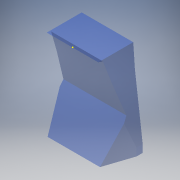
# Autodesk Inventor part: add
Saved by Autodesk Inventor 2018.1 (Build 221171000, 171)
## iProperties
Created: 2017-10-13
Part Number: add
Material: 一般
Document SubType Name: Modeling
Designer: kuwano
Density: 1 g/cm^3
Appearance: クリア - 青
Author: kuwano
Autodesk Inventor part; units mm, degrees
ref_plane "YZ Plane" through (0, 0, 0) normal (1, 0, 0) x (0, 1, 0)
ref_plane "XZ Plane" through (0, 0, 0) normal (0, 1, 0) x (-1, 0, 0)
ref_plane "XY Plane" through (0, 0, 0) normal (0, 0, 1) x (1, 0, 0)
sketch "スケッチ1" plane through (0, 0, 0) normal (0, 1, 0) x (-1, 0, 0)
  line L0 (341.5, 441.624) -> (-341.5, 441.624)
  line L1 (-341.5, 441.624) -> (-341.5, -441.624)
  line L2 (-341.5, -441.624) -> (341.5, -441.624)
  line L3 (341.5, -441.624) -> (341.5, 441.624)
  line L4 (0, -618.2736) -> (0, 618.2736) projected
  line L5 (478.1, 0) -> (-478.1, 0) projected
  point P0 (0, 0)
  point P1 (0, 441.624)
  point P2 (341.5, 0)
  dimension "d0" = 883.248
  dimension "d1" = 683
  constraints: 8 end point, 2 midpoint, 2 parallel, 2 point on line, 1 horizontal, 1 perpendicular
  measures "d0" distance of L2.end L0.start
  measures "d1" distance of L0.start L0.end
extrude "押し出し1" add sketch "スケッチ1" along normal blind 338.552
sketch "スケッチ2" plane through (0, 0, 0) normal (0, -1, 0) x (1, 0, 0)
  line L0 (-341.5, 441.624) -> (341.5, 441.624) projected
  line L1 (249.8123, 441.624) -> (266.1663, 220.287)
  line L2 (266.1663, 220.287) -> (341.5, -367.5482)
  line L3 (341.5, 441.624) -> (341.5, -441.624) projected
  line L4 (249.8123, 441.624) -> (341.5, 441.624)
  line L5 (341.5, 441.624) -> (341.5, -367.5482)
  line L6 (0, -782.4861) -> (0, 1603.5489) projected
  line L7 (-249.8123, 441.624) -> (-266.1663, 220.287)
  line L8 (-266.1663, 220.287) -> (-341.5, -367.5482)
  line L9 (-249.8123, 441.624) -> (-341.5, 441.624)
  line L10 (-341.5, 441.624) -> (-341.5, -367.5482)
  point P0 (0, 0)
  point P1 (0, 1262.6867)
  point P2 (-341.5, 441.624)
  constraints: 16 end point, 5 symmetric about line, 3 point on line, 1 horizontal, 1 perpendicular
extrude "押し出し2" cut sketch "スケッチ2" against normal through all
sketch "スケッチ3" plane through (-249.8123, 0, 441.624) normal (0, 0, 1) x (1, 0, 0)
  line L0 (0, 0) -> (499.6245, 0) projected
  line L1 (0, 0) -> (-91.6877, 278.2714)
  line L2 (-91.6877, 0) -> (-91.6877, 338.552) projected
  line L3 (-16.354, 0) -> (-91.6877, 0) projected
  line L4 (0, 0) -> (-91.6877, 0)
  line L5 (-91.6877, 0) -> (-91.6877, 278.2714)
  line L6 (249.8123, 0) -> (249.8123, -75.9213)
  line L7 (499.6245, 0) -> (0, 0)
  line L8 (499.6245, 0) -> (591.3123, 278.2714)
  line L9 (591.3123, 0) -> (591.3123, 338.552)
  line L10 (515.9785, 0) -> (591.3123, 0)
  line L11 (499.6245, 0) -> (591.3123, 0)
  line L12 (591.3123, 0) -> (591.3123, 278.2714)
  constraints: 20 end point, 6 symmetric about line, 2 point on line, 1 collinear, 1 perpendicular, 1 vertical
extrude "押し出し3" cut sketch "スケッチ3" against normal through all
sketch "スケッチ4" plane through (0, 0, 0) normal (1, 0, 0) x (0, 1, 0)
  line L0 (0, 441.624) -> (338.552, 441.624) projected
  line L1 (0, 441.624) -> (43.0995, 429.1359)
  line L2 (43.0995, 429.1359) -> (216.735, -84.6593)
  line L3 (216.735, -84.6593) -> (12.1682, -441.624)
  line L4 (0, -441.624) -> (278.2714, -441.624) projected
  line L5 (12.1682, -441.624) -> (0, -441.624)
  line L6 (0, -441.624) -> (0, 441.624)
  line L7 (0, 441.624) -> (338.552, 441.624)
  line L8 (338.552, 220.287) -> (338.552, -367.5482) projected
  line L9 (338.552, 441.624) -> (338.552, 220.287)
  line L10 (338.552, 220.287) -> (288.8719, 244.2421)
  line L11 (288.8719, 244.2421) -> (177.502, 390.1926)
  line L12 (177.502, 390.1926) -> (43.0995, 429.1359)
  point P0 (0, 0)
  constraints: 20 end point, 2 collinear, 1 perpendicular, 1 point on line, 1 vertical
extrude "押し出し5" cut sketch "スケッチ4" along normal through all both and the other way through all contours L0 L9 L10 L11 L12 L1
